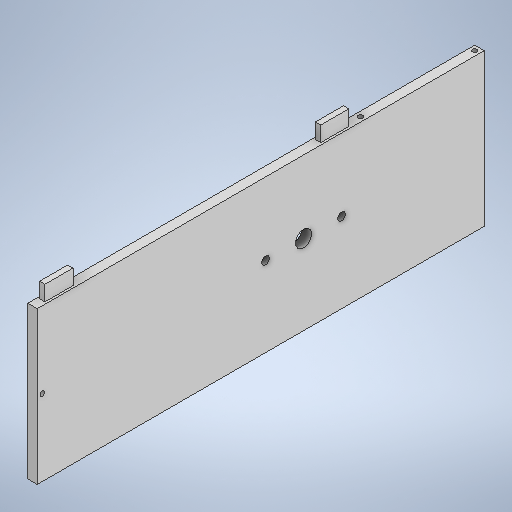
# Autodesk Inventor part: chassis_côté
Saved by Autodesk Inventor 2026.2 (Build 302298010, 298A)
## iProperties
Created: 2026-03-16
Part Number: chassis_côté
Material: Générique
Document SubType Name: Modeling
Designer: genon
Density: 1 g/cm^3
Appearance: Par défaut
Author: genon
Autodesk Inventor part; units mm, degrees
ref_plane "YZ Plane" through (0, 0, 0) normal (1, 0, 0) x (0, 1, 0)
ref_plane "XZ Plane" through (0, 0, 0) normal (0, 1, 0) x (-1, 0, 0)
ref_plane "XY Plane" through (0, 0, 0) normal (0, 0, 1) x (1, 0, 0)
sketch "Esquisse1" plane through (0, 0, 0) normal (1, 0, 0) x (0, 1, 0)
  line L0 (0, 0) -> (80, 0)
  line L1 (80, 0) -> (80, -200)
  line L2 (80, -200) -> (0, -200)
  line L3 (0, -200) -> (0, 0)
  dimension "d0" = 80
  dimension "d1" = 200
  constraints: 8 end point, 2 parallel, 1 horizontal, 1 perpendicular
  measures "d0" distance of L1.end L2.end
  measures "d1" distance of L0.end L1.end
extrude "Extrusion1" add sketch "Esquisse1" along normal blind 5
sketch "Esquisse7" plane through (5, 0, 0) normal (1, 0, 0) x (0, 0, -1)
  line L0 (0, 0) -> (100, 0)
  line L1 (0, 0) -> (200, 0) projected
  line L2 (100, 0) -> (180, 0) construction
  line L3 (100, 80) -> (100, 10)
  line L4 (100, 80) -> (170, 80) construction
  line L5 (120, 42) -> (80, 42)
  dimension "d50" = 100
  dimension "d54" = 90
  dimension "d80" = 40
  constraints: 10 end point, 3 horizontal, 1 coincident, 1 midpoint, 1 perpendicular
  measures "d50" distance of L0.start L0.end
  measures "d54" angle of L3 L4
  measures "d80" distance of L5.start L5.end
hole "Perçage6" at (5, 42, -120) at (5, 42, -80) direction (-1, 0, 0) diameter 4.134 end through all thread size "M5x0.8" class "6H" standard "ISO Metric profile"
sketch "Esquisse8" plane through (5, 0, 0) normal (1, 0, 0) x (0, 0, -1)
  circle A0 centre (80, 42) radius 2.067 projected
  line L0 (80, 42) -> (100, 42)
  point P0 (0, 0)
  constraints: 2 end point, 1 horizontal
hole "Perçage7" at (5, 42, -100) direction (-1, 0, 0) diameter 8.5 end through all
sketch "Esquisse9" plane through (0, 0, 0) normal (0, 0, 1) x (1, 0, 0)
  line L0 (0, 80) -> (0, 0) projected
  line L1 (0, 0) -> (5, 0) projected
  line L2 (5, 80) -> (5, 0) projected
  line L3 (0, 80) -> (5, 80) projected
extrude "Extrusion2" add sketch "Esquisse9" along normal blind 40
sketch "Esquisse5" plane through (0, 80, 0) normal (0, 1, 0) x (1, 0, 0)
  line L0 (0, 0) -> (5, 0) projected
  line L1 (2.5, 0) -> (5, 0) construction
  line L2 (0, 200) -> (0, 0) projected
  line L3 (0, 200) -> (5, 200) projected
  line L4 (0, 200) -> (0, 132.45)
  line L5 (0, 132.45) -> (2.5, 132.45)
  point P0 (2.5, 197.5)
  point P1 (0, -40)
  point P2 (2.5, 200)
  dimension "d84" = 2.5
  dimension "d85" = 2.5
  dimension "d86" = 67.55
  constraints: 6 end point, 2 midpoint, 1 coincident, 1 horizontal, 1 perpendicular, 1 point on line
  measures "d84" distance of point (2.5, 200) point (2.5, 197.5)
  measures "d85" distance from line of L2 point (2.5, 197.5)
  measures "d86" distance of L2.start L4.end
hole "Perçage4" at (2.5, 80, -197.5) at (2.5, 80, -132.45) direction (0, -1, 0) diameter 2.459 depth 15 thread size "M3x0.5" class "6H" standard "ISO Metric profile"
sketch "Esquisse4" plane through (0, 0, -200) normal (0, -1, 0) x (1, 0, 0)
  line L0 (0, 0) -> (0, 200) projected
  line L1 (5, 200) -> (5, 0) projected
  line L2 (5, 240) -> (0, 240) projected
  line L3 (0, 240) -> (2.5, 240)
  line L4 (2.5, 237.5) -> (2.5, 240)
  line L5 (0, 240) -> (0, 120)
  line L6 (0, 0) -> (5, 0) projected
  line L7 (0, 120) -> (2.5, 120)
  point P0 (2.5, 2.5)
  point P1 (2.5, 0)
  dimension "d87" = 120
  dimension "d88" = 2.5
  dimension "d89" = 2.5
  constraints: 8 end point, 2 coincident, 2 midpoint, 1 horizontal, 1 perpendicular, 1 point on line
  measures "d87" distance of L2.end L5.end
  measures "d88" distance from line of L0 point (2.5, 2.5)
  measures "d89" distance of point (2.5, 2.5) point (2.5, 0)
hole "Perçage3" at (2.5, 0, -197.5) at (2.5, 0, 37.5) at (2.5, 0, -80) direction (0, 1, 0) diameter 2.459 depth 15 thread size "M3x0.5" class "6H" standard "ISO Metric profile"
sketch "Esquisse3" plane through (5, 0, 0) normal (1, 0, 0) x (0, 0, -1)
  line L0 (0, 0) -> (200, 0) projected
  line L1 (-39.8826, 0) -> (-37.3826, 0)
  line L2 (-37.3826, 0) -> (-37.3826, 40)
  point P0 (197.5, 40)
  dimension "d90" = 2.5
  dimension "d91" = 40
  constraints: 4 end point, 1 coincident, 1 horizontal, 1 perpendicular
  measures "d90" distance of L1.start L1.end
  measures "d91" distance of L1.end L2.end
hole "Perçage2" at (5, 40, -197.5) at (5, 40, 37.3826) direction (-1, 0, 0) diameter 2.459 end through all thread size "M3x0.5" class "6H" standard "ISO Metric profile"
sketch "Esquisse10" plane through (0, 80, -200) normal (0, 1, 0) x (1, 0, 0)
  line L0 (5, -240) -> (0, -240) projected
  line L1 (2.5, -240) -> (2.5, -234.9)
  line L2 (2.5, -234.9) -> (3.9, -234.9)
  line L3 (2.5, -234.9) -> (1.1, -234.9)
  line L4 (1.1, -234.9) -> (1.1, -220.1)
  line L5 (1.1, -220.1) -> (3.9, -220.1)
  line L6 (3.9, -220.1) -> (3.9, -234.9)
  line L7 (0, -240) -> (0, -89.9)
  line L8 (0, 0) -> (0, -240) projected
  line L9 (0, -89.9) -> (1.1, -89.9)
  line L10 (1.1, -89.9) -> (3.9, -89.9)
  line L11 (3.9, -89.9) -> (3.9, -75.1)
  line L12 (3.9, -75.1) -> (1.1, -75.1)
  line L13 (1.1, -75.1) -> (1.1, -89.9)
  point P0 (0, -200)
  dimension "d92" = 5.1
  dimension "d93" = 1.4
  dimension "d94" = 1.4
  dimension "d95" = 14.8
  dimension "d96" = 150.1
  dimension "d97" = 1.1
  dimension "d98" = 14.8
  dimension "d99" = 2.8
  constraints: 24 end point, 8 perpendicular, 2 point on line, 1 horizontal, 1 midpoint, 1 vertical
  measures "d92" distance of L1.start L1.end
  measures "d93" distance of L1.end L2.end
  measures "d94" distance of L1.end L3.end
  measures "d95" distance of L3.end L4.end
  measures "d96" distance of L0.end L7.end
  measures "d97" distance of L7.end L9.end
  measures "d98" distance of L10.end L11.end
  measures "d99" distance of L11.end L12.end
extrude "Extrusion3" add sketch "Esquisse10" along normal blind 8
sketch "Esquisse11" plane through (5, 0, 0) normal (1, 0, 0) x (0, 0, -1)
  line L0 (200, 80) -> (-40, 80) projected
  line L1 (200, 0) -> (-40, 0) projected
  line L2 (200, 80) -> (195, 80)
  line L3 (195, 80) -> (195, 0)
  line L4 (195, 0) -> (200, 0)
  line L5 (200, 0) -> (200, 80)
  point P0 (0, 0)
  dimension "d102" = 5
  constraints: 8 end point, 2 parallel, 1 horizontal, 1 perpendicular, 1 point on line
  measures "d102" distance of L4.end L3.end
extrude "Extrusion4" cut sketch "Esquisse11" against normal blind 8
sketch "Esquisse12" plane through (0, 80, 40) normal (0, 1, 0) x (1, 0, 0)
  line L0 (0, 235) -> (0, 0) projected
  line L1 (0, 235) -> (2.5, 235)
  line L2 (0, 235) -> (5, 235) projected
  line L3 (2.5, 235) -> (2.5, 232.5)
  point P0 (0, 40)
  dimension "d105" = 2.5
  dimension "d106" = 2.5
  constraints: 4 end point, 1 coincident, 1 midpoint, 1 perpendicular
  measures "d105" distance of L0.start L1.end
  measures "d106" distance of L1.end L3.end
hole "Perçage8" at (2.5, 80, -192.5) direction (0, -1, 0) diameter 2.459 depth 15 thread size "M3x0.5" class "6H" standard "ISO Metric profile"
sketch "Esquisse13" plane through (0, 0, 40) normal (0, -1, 0) x (1, 0, 0)
  line L0 (0, -235) -> (0, 0) projected
  line L1 (0, -235) -> (2.5, -235)
  line L2 (5, -235) -> (0, -235) projected
  circle A0 centre (2.5, -232.5) radius 1.2295 projected
  point P0 (0, -40)
  constraints: 2 end point, 1 coincident, 1 midpoint
hole "Perçage9" at (2.5, 0, -192.5) direction (0, 1, 0) diameter 2.459 depth 15 thread size "M3x0.5" class "6H" standard "ISO Metric profile"
